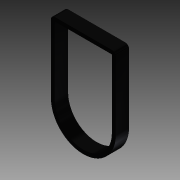
# Autodesk Inventor part: ZIP TIE GANTRY BEARING
Saved by Autodesk Inventor 2013 (Build 170138000, 138)
## iProperties
Created: 2014-06-21
Part Number: ZIP TIE GANTRY BEARING
Material: Generic
Document SubType Name: Modeling
Designer: employee
Density: 1 g/cm^3
Author: employee
Autodesk Inventor part; units mm, degrees
ref_plane "YZ Plane" through (0, 0, 0) normal (1, 0, 0) x (0, 1, 0)
ref_plane "XZ Plane" through (0, 0, 0) normal (0, 1, 0) x (-1, 0, 0)
ref_plane "XY Plane" through (0, 0, 0) normal (0, 0, 1) x (1, 0, 0)
sketch "Sketch1" plane through (0, 0, 0) normal (0, 0, 1) x (1, 0, 0)
  line L0 (1.5, 0) -> (0, 0) construction
  line L1 (1.5, 5.715) -> (1.5, 0) construction
  line L2 (0, 5.715) -> (1.5, 5.715) construction
  line L3 (0, 5.715) -> (0, 0) construction
  line L4 (1.5, -5.715) -> (0, -5.715) construction
  line L5 (1.5, 0) -> (1.5, -5.715) construction
  line L6 (0, 0) -> (1.5, 0) construction
  line L7 (0, 0) -> (0, -5.715) construction
  line L8 (18, -5.715) -> (16.5, -5.715) construction
  line L9 (18, 0) -> (18, -5.715) construction
  line L10 (16.5, 0) -> (18, 0) construction
  line L11 (16.5, 0) -> (16.5, -5.715) construction
  line L12 (18, 0) -> (16.5, 0) construction
  line L13 (18, 5.715) -> (18, 0) construction
  line L14 (16.5, 5.715) -> (18, 5.715) construction
  line L15 (16.5, 5.715) -> (16.5, 0) construction
  circle A0 centre (9, -12.2102) radius 7.5 construction
  line L16 (1.5, 5.715) -> (1.5, -12.2102)
  line L17 (16.5, 5.715) -> (16.5, -12.2102)
  arc A1 (1.5, -12.2102) -> (16.5, -12.2102) centre (9, -12.2102) ccw
  line L18 (1.5, 5.715) -> (16.5, 5.715)
  line L19 (17.5, 6.715) -> (17.5, -12.2102)
  arc A2 (0.5, -12.2102) -> (17.5, -12.2102) centre (9, -12.2102) ccw
  line L20 (0.5, -12.2102) -> (0.5, 6.715)
  line L21 (0.5, 6.715) -> (17.5, 6.715)
  dimension "d0" = 1
  constraints: 12 end point, 6 point on circle, 3 tangent, 2 centre point, 2 perpendicular, 1 point on line, 3 other
  measures "d0" distance between parallel lines of L21 L18
extrude "Extrusion1" add sketch "Sketch1" along normal blind 3.5
fillet "Fillet1" radius 1 2 edges at (0.5, 6.715, 1.75) (17.5, 6.715, 1.75)
body "Solid1"
